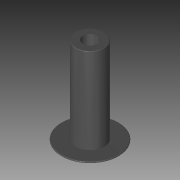
# Autodesk Inventor part: GripFinal
Saved by Autodesk Inventor 2016 (Build 200138000, 138)
## iProperties
Created: 2013-08-12
Part Number: GripFinal
Material: Rubber
Document SubType Name: Modeling
Designer: Anthony
Density: 0.93 g/cm^3
Appearance: Rubber - Black - Version 1.1
Author: Anthony
Autodesk Inventor part; units mm, degrees
ref_plane "YZ Plane" through (0, 0, 0) normal (1, 0, 0) x (0, 1, 0)
ref_plane "XZ Plane" through (0, 0, 0) normal (0, 1, 0) x (-1, 0, 0)
ref_plane "XY Plane" through (0, 0, 0) normal (0, 0, 1) x (1, 0, 0)
sketch "Sketch1" plane through (0, 0, 0) normal (0, 1, 0) x (-1, 0, 0)
  circle A0 centre (0, 0) radius 25.4
  dimension "d0" = 50.8
  constraints: 1 centre point, 1 coincident
  measures "d0" diameter of A0
extrude "Extrusion1" add sketch "Sketch1" along normal blind 2.8575
fillet "Fillet1" radius 0.635 1 edges at (25.4, 2.8575, 0)
fillet "Fillet2" radius 0.635 1 edges at (25.4, 0, 0)
sketch "Sketch2" plane through (0, 2.8575, 0) normal (0, 1, 0) x (1, 0, 0)
  circle A0 centre (0, 0) radius 24.765 projected
  circle A1 centre (0, 0) radius 6.35
  circle A2 centre (0, 0) radius 15.24
  dimension "d5" = 12.7
  dimension "d6" = 30.48
  constraints: 2 centre point, 2 coincident
  measures "d5" diameter of A1
  measures "d6" diameter of A2
extrude "Extrusion2" add sketch "Sketch2" along normal blind 128.5875 contours A2
fillet "Fillet3" radius 0.635 1 edges at (-15.24, 131.445, 0)
sketch "Sketch5" plane through (0, 0, 0) normal (0, -1, 0) x (1, 0, 0)
  circle A0 centre (0, 0) radius 24.765 projected
  circle A1 centre (0, 0) radius 6.35
  dimension "d34" = 12.7
  constraints: 1 centre point, 1 coincident
  measures "d34" diameter of A1
extrude "Extrusion4" cut sketch "Sketch5" against normal blind 1.27 contours A1
body "Solid1"
